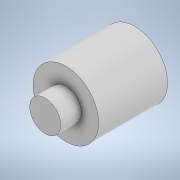
# Autodesk Inventor part: Marker Plunger
Saved by Autodesk Inventor 2022.2 (Build 262287010, 287A)
## iProperties
Created: 2022-02-25
Part Number: Marker Plunger
Material: ABS Plastic
Document SubType Name: Modeling
Designer: smiku
Density: 1.06 g/cm^3
Appearance: Smooth - Light Gray
Author: smiku
Autodesk Inventor part; units mm, degrees
ref_plane "YZ Plane" through (0, 0, 0) normal (1, 0, 0) x (0, 1, 0)
ref_plane "XZ Plane" through (0, 0, 0) normal (0, 1, 0) x (-1, 0, 0)
ref_plane "XY Plane" through (0, 0, 0) normal (0, 0, 1) x (1, 0, 0)
sketch "Sketch1" plane through (0, 0, 0) normal (0, 0, 1) x (1, 0, 0)
  circle A0 centre (0, 0) radius 4.5
  circle A1 centre (0, 0) radius 9.5
  dimension "d0" = 9
  dimension "d1" = 19
  constraints: 2 centre point, 2 coincident
  measures "d0" diameter of A0
  measures "d1" diameter of A1
extrude "Extrusion1" add sketch "Sketch1" against normal blind 20 contours A0 | A1
extrude "Extrusion2" add sketch "Sketch1" along normal blind 6 contours A0
shell "Shell1" thickness 1.2 removed faces 1 at (2.3703, -2.0999, -20)
chamfer "Chamfer1" distance 5 angle 45 1 edges at (-8.3, 0, -1.2)
body "Solid1"
